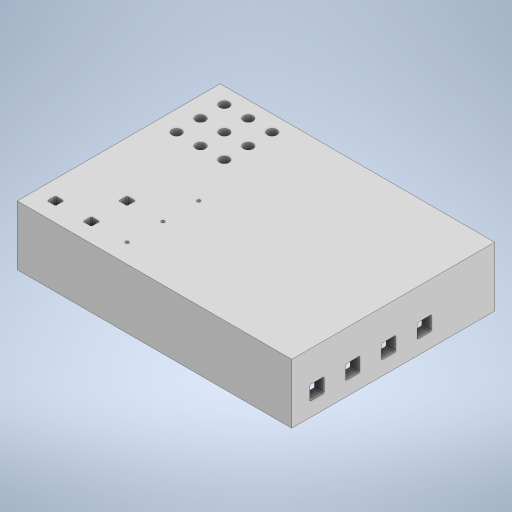
# Autodesk Inventor part: BreakoutBox
Saved by Autodesk Inventor 2023 (Build 270158000, 158)
## iProperties
Created: 2023-04-03
Part Number: BreakoutBox
Material: Generic
Document SubType Name: Modeling
Designer: yousefi
Density: 1 g/cm^3
Appearance: Default
Author: yousefi
Autodesk Inventor part; units mm, degrees
ref_plane "YZ Plane" through (0, 0, 0) normal (1, 0, 0) x (0, 1, 0)
ref_plane "XZ Plane" through (0, 0, 0) normal (0, 1, 0) x (-1, 0, 0)
ref_plane "XY Plane" through (0, 0, 0) normal (0, 0, 1) x (1, 0, 0)
sketch "main box1" plane through (0, 0, 0) normal (0, 1, 0) x (-1, 0, 0)
  line L0 (11.2873, -1.2021) -> (241.2873, -1.2021)
  line L1 (241.2873, -1.2021) -> (241.2873, -171.2021)
  line L2 (241.2873, -171.2021) -> (11.2873, -171.2021)
  line L3 (11.2873, -171.2021) -> (11.2873, -1.2021)
  point P0 (0, 0)
  dimension "d2" = 230
  dimension "d3" = 170
  constraints: 8 end point, 2 parallel, 1 horizontal, 1 perpendicular
  measures "d2" distance of L1.end L2.end
  measures "d3" distance of L0.end L1.end
extrude "Main box" add sketch "main box1" along normal blind 50
sketch "Ethernet1" plane through (-11.2873, 0, -1.2021) normal (1, 0, 0) x (0, 0, -1)
  line L0 (16, 24) -> (26, 24)
  line L1 (27, 23) -> (27, 13)
  line L2 (26, 12) -> (16, 12)
  line L3 (15, 13) -> (15, 23)
  line L4 (0, 0) -> (170, 0) projected
  line L5 (0, 0) -> (0, 50) projected
  arc A0 (16, 24) -> (15, 23) centre (16, 23) ccw
  arc A1 (15, 13) -> (16, 12) centre (16, 13) ccw
  arc A2 (26, 12) -> (27, 13) centre (26, 13) ccw
  arc A3 (27, 23) -> (26, 24) centre (26, 23) ccw
  line L6 (46, 24) -> (56, 24)
  line L7 (57, 23) -> (57, 13)
  line L8 (56, 12) -> (46, 12)
  line L9 (45, 13) -> (45, 23)
  arc A4 (46, 24) -> (45, 23) centre (46, 23) ccw
  arc A5 (45, 13) -> (46, 12) centre (46, 13) ccw
  arc A6 (56, 12) -> (57, 13) centre (56, 13) ccw
  arc A7 (57, 23) -> (56, 24) centre (56, 23) ccw
  arc A8 (76, 24) -> (75, 23) centre (76, 23) ccw
  arc A9 (75, 13) -> (76, 12) centre (76, 13) ccw
  line L10 (76, 24) -> (86, 24)
  arc A10 (87, 23) -> (86, 24) centre (86, 23) ccw
  line L11 (87, 23) -> (87, 13)
  line L12 (86, 12) -> (76, 12)
  arc A11 (86, 12) -> (87, 13) centre (86, 13) ccw
  line L13 (75, 13) -> (75, 23)
  arc A12 (106, 24) -> (105, 23) centre (106, 23) ccw
  line L14 (105, 13) -> (105, 23)
  arc A13 (105, 13) -> (106, 12) centre (106, 13) ccw
  line L15 (106, 24) -> (116, 24)
  line L16 (116, 12) -> (106, 12)
  arc A14 (117, 23) -> (116, 24) centre (116, 23) ccw
  line L17 (117, 23) -> (117, 13)
  arc A15 (116, 12) -> (117, 13) centre (116, 13) ccw
  point P0 (-1.2021, 0)
  point P1 (15, 24)
  point P2 (27, 12)
  point P3 (27, 24)
  point P4 (15, 12)
  point P5 (45, 24)
  point P6 (57, 12)
  point P7 (57, 24)
  point P8 (45, 12)
  point P9 (0, 25)
  point P10 (75, 24)
  point P11 (87, 24)
  point P12 (87, 12)
  point P13 (75, 12)
  point P14 (105, 24)
  point P15 (105, 12)
  point P16 (117, 24)
  point P17 (117, 12)
  dimension "d6" = 12
  dimension "d7" = 12
  dimension "d98" = 12
  dimension "d99" = 15
  dimension "d100" = 1
  dimension "d103" = 1
  dimension "d104" = 45
  dimension "d107" = 1
  dimension "d110" = 1
  dimension "d111" = 75
  dimension "d112" = 105
  constraints: 32 end point, 32 point on circle, 32 point on line, 32 tangent, 16 centre point, 12 equal radius, 9 collinear, 8 parallel, 4 horizontal, 4 perpendicular, 1 midpoint
  measures "d6" distance of point (27, 12) point (15, 12)
  measures "d7" distance of point (27, 24) point (27, 12)
  measures "d98" distance between parallel lines of L2 L4
  measures "d99" distance between parallel lines of L5 L3
  measures "d100" radius of A0
  measures "d103" radius of A4
  measures "d104" distance from line of point (0, 25) L9
  measures "d107" radius of A8
  measures "d110" radius of A12
  measures "d111" distance between parallel lines of L5 L13
  measures "d112" distance between parallel lines of L14 L5
extrude "Ethernet" cut sketch "Ethernet1" against normal blind 20
sketch "wheel 4 port connection" plane through (0, 50, 0) normal (0, 1, 0) x (1, 0, 0)
  line L0 (-222.7873, 20.7021) -> (-227.7873, 20.7021)
  line L1 (-228.7873, 19.7021) -> (-228.7873, 14.7021)
  line L2 (-227.7873, 13.7021) -> (-222.7873, 13.7021)
  line L3 (-221.7873, 14.7021) -> (-221.7873, 19.7021)
  line L4 (-241.2873, 171.2021) -> (-241.2873, 1.2021) projected
  line L5 (-241.2873, 1.2021) -> (-11.2873, 1.2021) projected
  arc A0 (-227.7873, 20.7021) -> (-228.7873, 19.7021) centre (-227.7873, 19.7021) ccw
  arc A1 (-221.7873, 19.7021) -> (-222.7873, 20.7021) centre (-222.7873, 19.7021) ccw
  arc A2 (-222.7873, 13.7021) -> (-221.7873, 14.7021) centre (-222.7873, 14.7021) ccw
  arc A3 (-228.7873, 14.7021) -> (-227.7873, 13.7021) centre (-227.7873, 14.7021) ccw
  point P0 (0, 0)
  point P1 (-221.7873, 20.7021)
  point P2 (-228.7873, 13.7021)
  point P3 (-228.7873, 20.7021)
  point P4 (-221.7873, 13.7021)
  dimension "d22" = 7
  dimension "d23" = 7
  dimension "d76" = 12.5
  dimension "d77" = 12.5
  dimension "d113" = 1
  constraints: 8 end point, 8 point on circle, 8 point on line, 8 tangent, 4 centre point, 3 equal radius, 2 parallel, 1 horizontal, 1 perpendicular
  measures "d22" distance of point (-221.787, 13.702) point (-228.787, 13.702)
  measures "d23" distance of point (-228.787, 13.702) point (-228.787, 20.702)
  measures "d76" distance between parallel lines of L1 L4
  measures "d77" distance between parallel lines of L5 L2
  measures "d113" radius of A0
extrude "wheel" cut sketch "wheel 4 port connection" against normal blind 20
sketch "Motor left 4 port connection" plane through (0, 50, 0) normal (0, 1, 0) x (1, 0, 0)
  line L0 (-192.7873, 20.7021) -> (-197.7873, 20.7021)
  line L1 (-198.7873, 19.7021) -> (-198.7873, 14.7021)
  line L2 (-197.7873, 13.7021) -> (-192.7873, 13.7021)
  line L3 (-191.7873, 14.7021) -> (-191.7873, 19.7021)
  line L4 (-241.2873, 1.2021) -> (-11.2873, 1.2021) projected
  line L5 (-221.7873, 19.7021) -> (-221.7873, 14.7021) projected
  arc A0 (-191.7873, 19.7021) -> (-192.7873, 20.7021) centre (-192.7873, 19.7021) ccw
  arc A1 (-192.7873, 13.7021) -> (-191.7873, 14.7021) centre (-192.7873, 14.7021) ccw
  arc A2 (-198.7873, 14.7021) -> (-197.7873, 13.7021) centre (-197.7873, 14.7021) ccw
  arc A3 (-197.7873, 20.7021) -> (-198.7873, 19.7021) centre (-197.7873, 19.7021) ccw
  point P0 (0, 0)
  point P1 (-191.7873, 20.7021)
  point P2 (-198.7873, 13.7021)
  point P3 (-198.7873, 20.7021)
  point P4 (-191.7873, 13.7021)
  point P5 (-221.7873, 20.7021)
  point P6 (-221.7873, 13.7021)
  dimension "d26" = 7
  dimension "d27" = 7
  dimension "d78" = 12.5
  dimension "d79" = 23
  dimension "d114" = 1
  constraints: 8 end point, 8 point on circle, 8 point on line, 8 tangent, 4 centre point, 3 equal radius, 2 parallel, 1 horizontal, 1 perpendicular
  measures "d26" distance of point (-191.787, 13.702) point (-198.787, 13.702)
  measures "d27" distance of point (-198.787, 13.702) point (-198.787, 20.702)
  measures "d78" distance between parallel lines of L4 L2
  measures "d79" distance between parallel lines of L5 L1
  measures "d114" radius of A0
extrude "Motor left" cut sketch "Motor left 4 port connection" against normal blind 20
sketch "Motor right 4 port connection" plane through (0, 50, 0) normal (0, 1, 0) x (1, 0, 0)
  line L0 (-197.7873, 43.7021) -> (-192.7873, 43.7021)
  line L1 (-191.7873, 44.7021) -> (-191.7873, 49.7021)
  line L2 (-192.7873, 50.7021) -> (-197.7873, 50.7021)
  line L3 (-198.7873, 49.7021) -> (-198.7873, 44.7021)
  line L4 (-197.7873, 20.7021) -> (-192.7873, 20.7021) projected
  line L5 (-198.7873, 14.7021) -> (-198.7873, 19.7021) projected
  arc A0 (-197.7873, 50.7021) -> (-198.7873, 49.7021) centre (-197.7873, 49.7021) ccw
  arc A1 (-191.7873, 49.7021) -> (-192.7873, 50.7021) centre (-192.7873, 49.7021) ccw
  arc A2 (-192.7873, 43.7021) -> (-191.7873, 44.7021) centre (-192.7873, 44.7021) ccw
  arc A3 (-198.7873, 44.7021) -> (-197.7873, 43.7021) centre (-197.7873, 44.7021) ccw
  point P0 (0, 0)
  point P1 (-198.7873, 43.7021)
  point P2 (-191.7873, 50.7021)
  point P3 (-191.7873, 43.7021)
  point P4 (-198.7873, 50.7021)
  point P5 (-198.7873, 20.7021)
  point P6 (-191.7873, 20.7021)
  point P7 (-198.7873, 13.7021)
  dimension "d30" = 7
  dimension "d31" = 7
  dimension "d80" = 23
  dimension "d115" = 1
  constraints: 8 end point, 8 point on circle, 8 point on line, 8 tangent, 4 centre point, 3 equal radius, 2 parallel, 1 collinear, 1 horizontal, 1 perpendicular
  measures "d30" distance of point (-198.787, 50.702) point (-191.787, 50.702)
  measures "d31" distance of point (-191.787, 50.702) point (-191.787, 43.702)
  measures "d80" distance between parallel lines of L4 L0
  measures "d115" radius of A0
extrude "Motor right" cut sketch "Motor right 4 port connection" against normal blind 20
sketch "Sketch10" plane through (0, 50, 0) normal (0, 1, 0) x (1, 0, 0)
  circle A0 centre (-165.2873, 17.2021) radius 1.35
  line L0 (-241.2873, 1.2021) -> (-11.2873, 1.2021) projected
  circle A1 centre (-165.2873, 47.2021) radius 1.35
  circle A2 centre (-165.2873, 77.2021) radius 1.35
  line L1 (-165.2873, 17.2021) -> (-165.2873, 77.2021) construction
  line L2 (-192.7873, 13.7021) -> (-197.7873, 13.7021) construction
  line L3 (-222.7873, 13.7021) -> (-227.7873, 13.7021) construction
  line L4 (-191.7873, 19.7021) -> (-191.7873, 14.7021) construction
  line L5 (-191.7873, 17.2021) -> (-165.2873, 17.2021) construction
  point P0 (0, 0)
  point P1 (-191.7873, 13.7021)
  point P2 (-198.7873, 13.7021)
  point P3 (-195.2873, 13.7021)
  point P4 (-221.7873, 13.7021)
  point P5 (-228.7873, 13.7021)
  point P6 (-195.2873, 13.7021)
  point P7 (-225.2873, 13.7021)
  point P8 (-191.7873, 20.7021)
  dimension "d34" = 2.7
  dimension "d86" = 30
  dimension "d87" = 30
  dimension "d88" = 30
  constraints: 5 midpoint, 4 end point, 3 centre point, 2 equal radius, 1 perpendicular, 1 vertical
  measures "d34" diameter of A0
  measures "d86" distance of L1.start A1.centre
  measures "d87" distance of L1.end A1.centre
  measures "d88" horizontal distance of L1.start point (-195.287, 13.702)
extrude "PD" cut sketch "Sketch10" against normal blind 20
sketch "Power socket" plane through (0, 50, 0) normal (0, 1, 0) x (1, 0, 0)
  circle A0 centre (-224.2873, 117.7021) radius 4
  line L0 (-241.2873, 171.2021) -> (-241.2873, 1.2021) projected
  circle A1 centre (-224.2873, 137.7021) radius 4
  circle A2 centre (-224.2873, 157.7021) radius 4
  circle A3 centre (-204.2873, 157.7021) radius 4
  circle A4 centre (-204.2873, 137.7021) radius 4
  circle A5 centre (-204.2873, 117.7021) radius 4
  circle A6 centre (-184.2873, 157.7021) radius 4
  circle A7 centre (-184.2873, 137.7021) radius 4
  circle A8 centre (-184.2873, 117.7021) radius 4
  line L1 (-11.2873, 171.2021) -> (-241.2873, 171.2021) projected
  line L2 (-224.2873, 117.7021) -> (-224.2873, 157.7021) construction
  line L3 (-224.2873, 157.7021) -> (-184.2873, 157.7021) construction
  line L4 (-184.2873, 157.7021) -> (-184.2873, 117.7021) construction
  line L5 (-184.2873, 117.7021) -> (-224.2873, 117.7021) construction
  line L6 (-224.2873, 137.7021) -> (-184.2873, 137.7021) construction
  line L7 (-204.2873, 157.7021) -> (-204.2873, 117.7021) construction
  point P0 (0, 0)
  dimension "d43" = 8
  dimension "d90" = 17
  dimension "d94" = 13.5
  dimension "d95" = 20
  dimension "d96" = 20
  constraints: 12 end point, 9 centre point, 8 equal radius, 6 midpoint, 5 perpendicular, 3 coincident, 1 vertical
  measures "d43" diameter of A0
  measures "d90" distance from line of L0 L2.start
  measures "d94" distance from line of L1 A2.centre
  measures "d95" distance of L6.start A2.centre
  measures "d96" distance of L7.start A2.centre
extrude "Power" cut sketch "Power socket" against normal blind 20
sketch "Sketch22" plane through (0, 0, 0) normal (0, -1, 0) x (1, 0, 0)
  line L0 (-19.2873, -9.2021) -> (-233.2873, -9.2021)
  line L1 (-233.2873, -9.2021) -> (-233.2873, -163.2021)
  line L2 (-233.2873, -163.2021) -> (-19.2873, -163.2021)
  line L3 (-19.2873, -163.2021) -> (-19.2873, -9.2021)
  line L4 (-241.2873, -1.2021) -> (-11.2873, -1.2021) projected
  line L5 (-11.2873, -171.2021) -> (-241.2873, -171.2021) projected
  line L6 (-11.2873, -1.2021) -> (-11.2873, -171.2021) projected
  line L7 (-241.2873, -171.2021) -> (-241.2873, -1.2021) projected
  point P0 (0, 0)
  dimension "d70" = 8
  dimension "d71" = 8
  dimension "d72" = 8
  dimension "d73" = 8
  constraints: 8 end point, 2 parallel, 1 horizontal, 1 perpendicular
  measures "d70" distance between parallel lines of L4 L0
  measures "d71" distance between parallel lines of L5 L2
  measures "d72" distance between parallel lines of L6 L3
  measures "d73" distance between parallel lines of L7 L1
extrude "Extrusion21" cut sketch "Sketch22" against normal blind 42 contours L3 L2 L1 L0
body "Solid1"
